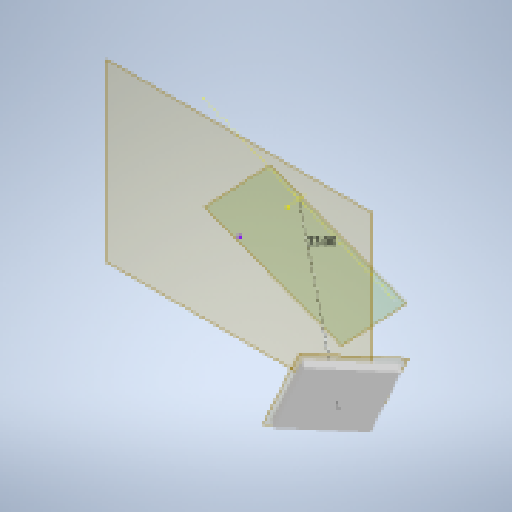
# Autodesk Inventor part: lustro
Saved by Autodesk Inventor 2025.1 (Build 291241020, 241B)
## iProperties
Created: 2024-10-13
Part Number: lustro
Material: Ogólny
Document SubType Name: Modeling
Designer: zychlix
Density: 1 g/cm^3
Appearance: Domyślna
Author: zychlix
Autodesk Inventor part; units mm, degrees
ref_plane "YZ Plane" through (0, 0, 0) normal (1, 0, 0) x (0, 1, 0)
ref_plane "XZ Plane" through (0, 0, 0) normal (0, 1, 0) x (-1, 0, 0)
ref_plane "XY Plane" through (0, 0, 0) normal (0, 0, 1) x (1, 0, 0)
ref_plane "Płaszczyzna konstrukcyjna1" through (0, 0, 13) normal (0, 0, 1) x (1, 0, 0)
sketch "Szkic2" plane through (0, 0, 13) normal (0, 0, 1) x (1, 0, 0)
  point P0 (0, 0)
ref_plane "Płaszczyzna konstrukcyjna2" through (0, 0, 13) normal (-0.3820784, -0.9224189, -0.0562099) x (0, 0.0608247, -0.9981485)
sketch "Szkic3" plane through (0, 0, 13) normal (-0.3820784, -0.9224189, -0.0562099) x (0, 0.0608247, -0.9981485)
  line L0 (16.0297, 0) -> (-11.4737, 40.3276) construction
  line L1 (15.3925, 28.2071) -> (16.6668, -28.2071) construction
  point P0 (12.9759, 0.3021)
  point P1 (-9.1944, 36.9855)
  dimension "d2" = 33
  constraints: 2 end point, 1 point on line
  measures "d2" angle of L1 L0
ref_plane "Płaszczyzna konstrukcyjna7" through (34.1794, -14.6644, 21.3179) normal (0.7634769, -0.3493435, 0.5431962) x (0.4160804, 0.9093278, 0)
sketch "Szkic4" plane through (34.1794, -14.6644, 21.3179) normal (0.7634769, -0.3493435, 0.5431962) x (0.4160804, 0.9093278, 0)
  line L0 (-10.061, 9.7866) -> (9.939, 9.7866)
  line L1 (9.939, 9.7866) -> (9.939, -9.8769)
  line L2 (9.939, -9.8769) -> (-10.061, -9.8769)
  line L3 (-10.061, -9.8769) -> (-10.061, 9.7866)
  point P0 (-0.8866, 2.2985)
  dimension "d3" = 20
  constraints: 8 end point, 2 parallel, 1 horizontal, 1 perpendicular
  measures "d3" distance of L1.end L2.end
extrude "Wyciągnięcie proste2" add sketch "Szkic4" along normal blind 2
